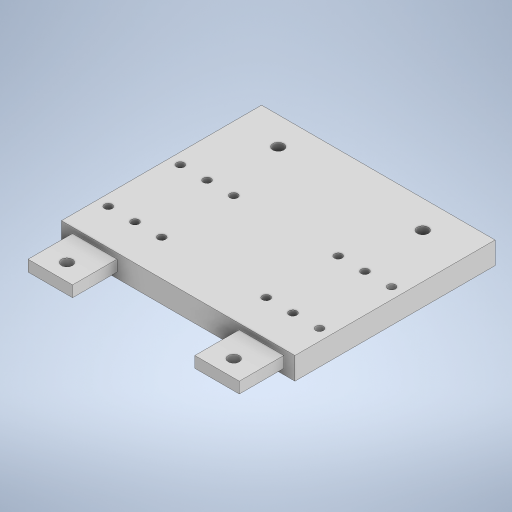
# Autodesk Inventor part: base_back
Saved by Autodesk Inventor 2023 (Build 270158000, 158)
## iProperties
Created: 2022-10-20
Part Number: base_back
Material: Genérico
Document SubType Name: Modeling
Designer: inigo
Density: 1 g/cm^3
Appearance: Valor por defecto
Author: inigo
Autodesk Inventor part; units mm, degrees
ref_plane "YZ Plane" through (0, 0, 0) normal (1, 0, 0) x (0, 1, 0)
ref_plane "XZ Plane" through (0, 0, 0) normal (0, 1, 0) x (-1, 0, 0)
ref_plane "XY Plane" through (0, 0, 0) normal (0, 0, 1) x (1, 0, 0)
sketch "Boceto1" plane through (0, 0, 0) normal (0, 1, 0) x (-1, 0, 0)
  line L0 (105, 90) -> (-105, 90)
  line L1 (-105, 90) -> (-105, -90)
  line L2 (-105, -90) -> (105, -90)
  line L3 (105, -90) -> (105, 90)
  line L4 (105, 90) -> (-105, -90) construction
  line L5 (-105, 90) -> (105, -90) construction
  point P0 (0, 0)
  dimension "d0" = 210
  dimension "d1" = 180
  constraints: 12 end point, 2 midpoint, 2 parallel, 1 horizontal, 1 perpendicular
  measures "d0" distance of L2.end L1.end
  measures "d1" distance of L1.end L0.end
extrude "Extrusión1" add sketch "Boceto1" along normal blind 20
sketch "Boceto2" plane through (0, 20, 0) normal (0, 1, 0) x (1, 0, 0)
  circle A0 centre (-95, -57.83) radius 3.5
  line L0 (-105, -65.43) -> (-37, -65.43)
  line L1 (-37, -65.43) -> (-37, 14.57)
  line L2 (-37, 14.57) -> (-105, 14.57)
  line L3 (-105, 14.57) -> (-105, -65.43)
  line L4 (-71, -65.43) -> (-71, -8.508)
  circle A1 centre (-71, -57.83) radius 3.5
  circle A2 centre (-47, -57.83) radius 3.5
  line L5 (-37, -25.43) -> (-48.2072, -25.43)
  circle A3 centre (-47, 6.97) radius 3.5
  circle A4 centre (-71, 6.97) radius 3.5
  circle A5 centre (-95, 6.97) radius 3.5
  line L6 (0, 0) -> (0, 47.1145)
  circle A6 centre (95, -57.83) radius 3.5
  line L7 (105, -65.43) -> (37, -65.43)
  line L8 (37, -65.43) -> (37, 14.57)
  line L9 (37, 14.57) -> (105, 14.57)
  line L10 (105, 14.57) -> (105, -65.43)
  line L11 (71, -65.43) -> (71, -8.508)
  circle A7 centre (71, -57.83) radius 3.5
  circle A8 centre (47, -57.83) radius 3.5
  line L12 (37, -25.43) -> (48.2072, -25.43)
  circle A9 centre (47, 6.97) radius 3.5
  circle A10 centre (71, 6.97) radius 3.5
  circle A11 centre (95, 6.97) radius 3.5
  circle A12 centre (-65, 65) radius 5
  circle A13 centre (65, 65) radius 5
  circle A14 centre (65, 65) radius 5
  line L13 (0, 0) -> (210, 0)
  line L14 (0, 0) -> (210, 0)
  line L15 (210, 0) -> (105, 0)
  circle A15 centre (40, -25) radius 5
  circle A16 centre (0, -75) radius 10
  line L16 (-105, -90) -> (105, -90) projected
  dimension "d4" = 7
  dimension "d5" = 68
  dimension "d6" = 80
  dimension "d7" = 7.6
  dimension "d8" = 10
  dimension "d9" = 7
  dimension "d11" = 24
  dimension "d14" = 10
  dimension "d16" = 10
  dimension "d30" = 20
  dimension "d31" = 0
  dimension "d32" = 15
  constraints: 32 end point, 19 symmetric about line, 17 centre point, 3 horizontal, 3 midpoint, 2 parallel, 2 point on line, 2 vertical, 1 perpendicular, 11 other
  measures "d4" diameter of A0
  measures "d5" distance of L2.end L1.end
  measures "d6" distance of L1.end L0.end
  measures "d7" distance from line of L0 A0.centre
  measures "d8" distance from line of L3 A0.centre
  measures "d9" diameter of A1
  measures "d11" distance of A4.centre A5.centre
  measures "d14" diameter of A12
  measures "d16" diameter of A13
  measures "d30" diameter of A16
  measures "d31" distance from line of L6 A16.centre
  measures "d32" distance from line of L16 A16.centre
extrude "Extrusión2" cut sketch "Boceto2" against normal blind 20 contours A0 | A1 L4 | L4 A1 | A2 | A3 | A4 | A5 | A6 | A7 L11 | L11 A7 | A8 | A9 | A10 | A11 | A12 | A13
sketch "Boceto4" plane through (-105, 0, 90) normal (0, 0, 1) x (1, 0, 0)
  line L0 (10, 15) -> (50, 15)
  line L1 (50, 15) -> (50, 5)
  line L2 (50, 5) -> (10, 5)
  line L3 (10, 5) -> (10, 15)
  line L4 (10, 15) -> (50, 5) construction
  line L5 (50, 15) -> (10, 5) construction
  line L6 (0, 0) -> (0, 20) projected
  line L7 (0, 20) -> (210, 20) projected
  line L8 (105, 20) -> (105, 5.8224)
  line L9 (200, 15) -> (160, 15)
  line L10 (160, 15) -> (160, 5)
  line L11 (160, 5) -> (200, 5)
  line L12 (200, 5) -> (200, 15)
  line L13 (200, 15) -> (160, 5) construction
  line L14 (160, 15) -> (200, 5) construction
  point P0 (105, 0)
  point P1 (30, 10)
  point P2 (180, 10)
  dimension "d36" = 40
  dimension "d37" = 10
  dimension "d38" = 10
  constraints: 26 end point, 5 symmetric about line, 3 midpoint, 2 parallel, 1 horizontal, 1 perpendicular, 1 vertical
  measures "d36" distance of L1.end L2.end
  measures "d37" distance of L0.end L1.end
  measures "d38" distance between parallel lines of L6 L3
extrude "Extrusión4" add sketch "Boceto4" along normal blind 40
sketch "Boceto5" plane through (-95, 15, 90) normal (0, 1, 0) x (1, 0, 0)
  circle A0 centre (20, -25) radius 5
  line L0 (-10, 0) -> (200, 0) projected
  line L1 (95, 0) -> (95, -22.5331)
  circle A1 centre (170, -25) radius 5
  line L2 (40, -40) -> (0, -40) projected
  point P0 (95, 90)
  dimension "d41" = 10
  dimension "d54" = 15
  constraints: 2 centre point, 2 end point, 1 midpoint, 1 symmetric about line, 1 vertical, 1 other
  measures "d41" diameter of A0
  measures "d54" distance from line of L2 A0.centre
extrude "Extrusión5" cut sketch "Boceto5" against normal blind 40
